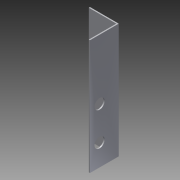
# Autodesk Inventor part: Limit Switch Bracket Shooter Front Right Corner
Saved by Autodesk Inventor 2014 SP1 (Build 180222100, 222)
## iProperties
Created: 2013-12-13
Part Number: Limit Switch Bracket Shooter Front Right Corner
Material: Aluminum 6061
Document SubType Name: Modeling
Designer: Moses
Density: 2.71 g/cm^3
Appearance: Aluminum - Flat
Mass: 5.91161 g
Surface Area: 57.2935 cm^2
Volume: 2.18141 cm^3
Author: Moses
Autodesk Inventor part; units mm, degrees
ref_plane "YZ Plane" through (0, 0, 0) normal (1, 0, 0) x (0, 1, 0)
ref_plane "XZ Plane" through (0, 0, 0) normal (0, 1, 0) x (-1, 0, 0)
ref_plane "XY Plane" through (0, 0, 0) normal (0, 0, 1) x (1, 0, 0)
sketch "Sketch1" plane through (0, 0, 0) normal (0, 1, 0) x (-1, 0, 0)
  line L0 (0, 0) -> (0, 19.05)
  line L1 (0, 19.05) -> (0.7937, 19.05)
  line L2 (0.7937, 19.05) -> (0.7938, 0.7937)
  line L3 (0.7938, 0.7937) -> (19.05, 0.7937)
  line L4 (19.05, 0.7937) -> (19.05, 0)
  line L5 (19.05, 0) -> (0, 0)
  dimension "d0" = 19.05
  dimension "d1" = 0.7937
  constraints: 12 end point, 3 horizontal, 3 vertical, 2 perpendicular
  measures "d0" distance of L0.start L0.end
  measures "d1" distance of L0.end L1.end
extrude "Extrusion1" add sketch "Sketch1" along normal blind 76.2
sketch "Sketch2" plane through (0, 0, 19.05) normal (1, 0, 0) x (0, 0, -1)
  line L0 (19.05, 0) -> (19.05, 76.2) projected
  line L1 (6.35, 36.5125) -> (6.35, 14.2875) construction
  circle A0 centre (6.35, 36.5125) radius 3.3782
  circle A1 centre (6.35, 14.2875) radius 3.3782
  line L2 (19.05, 0) -> (0, 0) projected
  dimension "d4" = 22.225
  dimension "d5" = 6.7564
  dimension "d16" = 12.7
  dimension "d17" = 14.2875
  constraints: 2 centre point, 2 coincident, 2 end point, 1 equal radius, 1 vertical
  measures "d4" distance of L1.start L1.end
  measures "d5" diameter of A0
  measures "d16" distance between parallel lines of L0 L1
  measures "d17" distance from line of L2 L1.end
extrude "Extrusion2" cut sketch "Sketch2" against normal through all
sketch "Sketch3" plane through (0, 0, 0) normal (0, 0, -1) x (-1, 0, 0)
  line L0 (0, 76.2) -> (19.05, 76.2) projected
  line L1 (0, 0) -> (0, 76.2) projected
  line L2 (16.65, 57.15) -> (6.35, 57.15) construction
  line L3 (6.35, 57.15) -> (6.35, 35.45) construction
  line L4 (6.35, 35.45) -> (16.65, 35.45) construction
  line L5 (16.65, 35.45) -> (16.65, 57.15) construction
  circle A0 centre (16.65, 35.45) radius 1.905
  circle A1 centre (6.35, 57.15) radius 1.905
  dimension "d9" = 3.81
  dimension "d10" = 21.7
  dimension "d11" = 10.3
  dimension "d12" = 19.05
  dimension "d13" = 6.35
  constraints: 8 end point, 2 centre point, 2 coincident, 2 parallel, 1 equal radius, 1 horizontal, 1 perpendicular
  measures "d9" diameter of A0
  measures "d10" distance of L4.end L2.start
  measures "d11" distance of L3.end L4.end
  measures "d12" distance between parallel lines of L0 L2
  measures "d13" distance between parallel lines of L1 L3
extrude "Extrusion3" cut sketch "Sketch3" against normal through all
body "Solid1"
